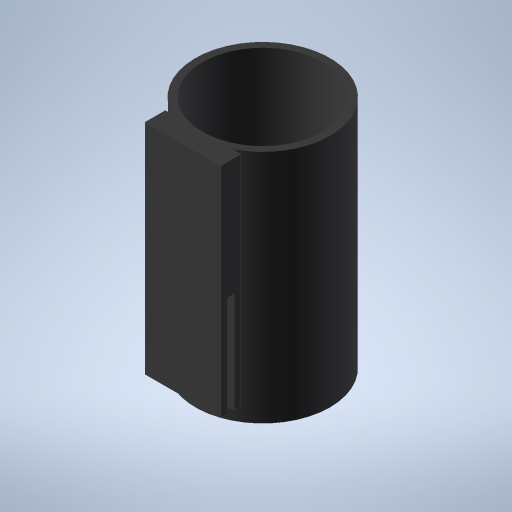
# Autodesk Inventor part: Part9
Saved by Autodesk Inventor 2023.2 (Build 272271030, 271C)
## iProperties
Created: 2024-03-23
Part Number: Part9
Material: Generic
Document SubType Name: Modeling
Designer: ryanv
Density: 1 g/cm^3
Appearance: Default
Author: ryanv
Autodesk Inventor part; units mm, degrees
ref_plane "YZ Plane" through (0, 0, 0) normal (1, 0, 0) x (0, 1, 0)
ref_plane "XZ Plane" through (0, 0, 0) normal (0, 1, 0) x (-1, 0, 0)
ref_plane "XY Plane" through (0, 0, 0) normal (0, 0, 1) x (1, 0, 0)
sketch "Sketch1" plane through (0, 0, 0) normal (0, 1, 0) x (-1, 0, 0)
  circle A0 centre (0, 0) radius 6.6
  dimension "d0" = 13.2
  constraints: 1 centre point, 1 coincident
  measures "d0" diameter of A0
extrude "Extrusion1" add sketch "Sketch1" along normal blind 20
sketch "Sketch3" plane through (0, 20, 0) normal (0, 1, 0) x (1, 0, 0)
  circle A0 centre (0, 0) radius 40
  dimension "d4" = 80
  constraints: 1 centre point, 1 coincident
  measures "d4" diameter of A0
extrude "Extrusion2" add sketch "Sketch3" along normal blind 140
sketch "Sketch4" plane through (0, 160, 0) normal (0, 1, 0) x (1, 0, 0)
  circle A0 centre (0, 0) radius 36
  circle A1 centre (0, 0) radius 40 projected
  dimension "d7" = 72
  constraints: 1 centre point, 1 coincident, 1 concentric
  measures "d7" diameter of A0
extrude "Extrusion3" cut sketch "Sketch4" against normal blind 130 contours A0
sketch "Sketch5" plane through (0, 0, 0) normal (0, -1, 0) x (1, 0, 0)
  circle A0 centre (0, 0) radius 5.3852
  circle A1 centre (0, 0) radius 6.6 projected
  constraints: 1 centre point, 1 coincident, 1 concentric
extrude "Extrusion4" cut sketch "Sketch5" against normal blind 130 contours A0
sketch "Sketch6" plane through (0, 160, 0) normal (0, 1, 0) x (1, 0, 0)
  line L0 (23, -36) -> (-22, -36)
  line L1 (-22, -36) -> (-22, -48)
  line L2 (-22, -48) -> (23, -48)
  line L3 (23, -48) -> (23, -36)
  point P0 (0, 0)
  constraints: 8 end point, 2 parallel, 1 horizontal, 1 perpendicular
extrude "Extrusion5" add sketch "Sketch6" against normal blind 130
sketch "Sketch7" plane through (0, 30, 0) normal (0, -1, 0) x (1, 0, 0)
  line L0 (-25, 44) -> (25, 44)
  line L1 (25, 44) -> (25, 40)
  line L2 (25, 40) -> (-25, 40)
  line L3 (-25, 40) -> (-25, 44)
  line L4 (23, 48) -> (-22, 48) projected
  point P0 (0, 0)
  dimension "d17" = 4
  constraints: 8 end point, 2 parallel, 1 horizontal, 1 perpendicular
  measures "d17" distance between parallel lines of L0 L4
extrude "Extrusion6" cut sketch "Sketch7" against normal blind 60
body "Solid1"
